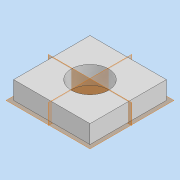
# Autodesk Inventor part: bearing3b
Saved by Autodesk Inventor 2022 (Build 260153000, 153)
## iProperties
Created: 2024-01-11
Part Number: bearing3b
Material: 一般
Document SubType Name: Modeling
Designer: ktamu
Density: 1 g/cm^3
Appearance: 既定
Author: ktamu
Autodesk Inventor part; units mm, degrees
sketch "スケッチ1" plane through (0, 0, 0) normal (0, 1, 0) x (-1, 0, 0)
  circle A0 centre (0, 0) radius 17.5
  line L0 (36, -36) -> (-36, -36)
  line L1 (-36, -36) -> (-36, 36)
  line L2 (-36, 36) -> (36, 36)
  line L3 (36, 36) -> (36, -36)
  line L4 (36, -36) -> (-36, 36) construction
  line L5 (-36, -36) -> (36, 36) construction
  dimension "d0" = 35
  dimension "d1" = 72
  dimension "d2" = 72
  constraints: 12 end point, 2 midpoint, 2 parallel, 1 centre point, 1 coincident, 1 horizontal, 1 perpendicular
  measures "d0" diameter of A0
  measures "d1" distance of L1.end L2.end
  measures "d2" distance of L0.end L1.end
extrude "押し出し1" add sketch "スケッチ1" along normal blind 17
